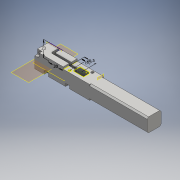
# Autodesk Inventor part: bas_de_fourche_gros_bloc
Saved by Autodesk Inventor 2016 (Build 200138000, 138)
## iProperties
Created: 2017-07-06
Part Number: bas_de_fourche_gros_bloc
Material: Generic
Document SubType Name: Modeling
Designer: mbouhier
Density: 1 g/cm^3
Appearance: Default
Author: mbouhier
Autodesk Inventor part; units mm, degrees
ref_plane "YZ Plane" through (0, 0, 0) normal (1, 0, 0) x (0, 1, 0)
ref_plane "XZ Plane" through (0, 0, 0) normal (0, 1, 0) x (-1, 0, 0)
ref_plane "XY Plane" through (0, 0, 0) normal (0, 0, 1) x (1, 0, 0)
sketch "Sketch1" plane through (0, 0, 0) normal (0, 1, 0) x (-1, 0, 0)
  line L0 (-10, 11.5) -> (10, 11.5)
  line L1 (10, 11.5) -> (10, -11.5)
  line L2 (10, -11.5) -> (-10, -11.5)
  line L3 (-10, -11.5) -> (-10, 11.5)
  line L4 (-10, 11.5) -> (10, -11.5) construction
  line L5 (10, 11.5) -> (-10, -11.5) construction
  point P0 (0, 0)
  dimension "d0" = 20
  dimension "d1" = 23
  constraints: 12 end point, 2 midpoint, 2 parallel, 1 horizontal, 1 perpendicular
  measures "d0" distance of L1.end L2.end
  measures "d1" distance of L0.end L1.end
extrude "Extrusion2" add sketch "Sketch1" against normal blind 20
ref_plane "Work Plane1" through (-10, 0, 0) normal (0, 0, 1) x (1, 0, 0)
ref_plane "Work Plane2" through (0, -2, 0) normal (0, 1, 0) x (1, 0, 0)
sketch "Sketch11" plane through (0, -2, 0) normal (0, 1, 0) x (1, 0, 0)
  point P0 (0, 0)
sketch "Sketch12" plane through (10, 0, 11.5) normal (1, 0, 0) x (0, 0, -1)
  line L0 (23, -20) -> (0, -20)
  line L1 (0, -20) -> (0, 0)
  line L2 (0, 0) -> (23, 0)
  line L3 (23, 0) -> (23, -20)
  point P0 (11.5, 0)
  dimension "d41" = 23
  dimension "d42" = 20
  constraints: 8 end point, 2 parallel, 1 horizontal, 1 perpendicular
  measures "d41" distance of L1.end L2.end
  measures "d42" distance of L0.end L1.end
extrude "Extrusion4" add sketch "Sketch12" along normal blind 22
sketch "Sketch13" plane through (32, 0, 11.5) normal (1, 0, 0) x (0, 0, -1)
  line L0 (23, 0) -> (23, -20) projected
  line L1 (23, -20) -> (3, -20)
  line L2 (3, -20) -> (3, 0)
  line L3 (3, 0) -> (23, 0)
  line L4 (23, 0) -> (23, -20)
  point P0 (11.5, 0)
  dimension "d45" = 20
  constraints: 8 end point, 2 parallel, 1 horizontal, 1 perpendicular
  measures "d45" distance of L1.end L2.end
extrude "Extrusion5" add sketch "Sketch13" along normal blind 120
sketch "Sketch26" plane through (32, -20, 8.5) normal (0, 0, 1) x (1, 0, 0)
  line L0 (8, 15) -> (23, 15)
  line L1 (23, 15) -> (23, 5)
  line L2 (23, 5) -> (8, 5)
  line L3 (8, 5) -> (8, 15)
  line L4 (0, 20) -> (120, 20) projected
  line L5 (0, 0) -> (120, 0) projected
  point P0 (-32, 20)
  dimension "d91" = 15
  dimension "d92" = 10
  dimension "d93" = 5
  dimension "d94" = 5
  constraints: 8 end point, 2 parallel, 1 horizontal, 1 perpendicular
  measures "d91" distance of L1.end L2.end
  measures "d92" distance of L0.end L1.end
  measures "d93" distance between parallel lines of L0 L4
  measures "d94" distance between parallel lines of L5 L2
extrude "Extrusion12" cut sketch "Sketch26" against normal blind 15
sketch "Sketch28" plane through (10, 0, -11.5) normal (0, 0, -1) x (-1, 0, 0)
  line L0 (-22, 0) -> (-22, -20) projected
  line L1 (20, -20) -> (-142, -20) projected
  line L2 (-22, 0) -> (-142, 0) projected
  point P0 (10, 0)
  point P1 (-27, -17)
  point P2 (-46, -3)
  dimension "d101" = 19
  dimension "d102" = 5
  dimension "d103" = 3
  dimension "d104" = 3
  measures "d101" horizontal distance of point (-46, -3) point (-27, -17)
  measures "d102" distance from line of L0 point (-27, -17)
  measures "d103" distance from line of L1 point (-27, -17)
  measures "d104" distance from line of L2 point (-46, -3)
hole "Hole3" at (56, -3, -11.5) at (37, -17, -11.5) direction (0, 0, 1) diameter 3.5 end through all counterbore diameter 5.5 counterbore depth 4
sketch "Sketch29" plane through (0, -20, 0) normal (0, -1, 0) x (1, 0, 0)
  line L0 (10, 11.5) -> (-10, 11.5) projected
  line L1 (10, -11.5) -> (10, 11.5) projected
  line L2 (-10, -11.5) -> (152, -11.5) projected
  line L3 (-10, 11.5) -> (-10, -11.5) projected
  point P0 (0, 0)
  point P1 (6.5, -8)
  point P2 (-6.5, 8)
  dimension "d112" = 3.5
  dimension "d113" = 3.5
  dimension "d128" = 3.5
  dimension "d129" = 3.5
  measures "d112" distance from line of L1 point (6.5, -8)
  measures "d113" distance from line of point (-6.5, 8) L3
  measures "d128" distance from line of L2 point (6.5, -8)
  measures "d129" distance from line of L0 point (-6.5, 8)
hole "Hole4" at (-6.5, -20, 8) at (6.5, -20, -8) direction (0, 1, 0) diameter 3.7 end through all counterbore diameter 6 counterbore depth 4
sketch "Sketch38" plane through (0, -20, 0) normal (0, -1, 0) x (1, 0, 0)
  circle A0 centre (-6.5, 8) radius 3 projected
  circle A1 centre (6.5, -8) radius 3 projected
  circle A2 centre (-6.5, 8) radius 3 projected
  circle A3 centre (6.5, -8) radius 3 projected
  line L0 (-10, 11.5) -> (32, 11.5) projected
  line L1 (-10, 11.5) -> (-10, -11.5) projected
  line L2 (-10, -11.5) -> (152, -11.5) projected
  line L3 (152, 8.5) -> (152, -11.5) projected
  line L4 (32, 8.5) -> (152, 8.5) projected
  line L5 (32, 11.5) -> (32, 8.5) projected
  circle A4 centre (-6.5, 8) radius 3 projected
  line L6 (-10, 11.5) -> (-10, -11.5) projected
  line L7 (-10, -11.5) -> (152, -11.5) projected
  line L8 (3.5, -11.5) -> (3.5, -8)
  circle A5 centre (6.5, -8) radius 3 projected
  line L9 (9.5, -8) -> (9.5, -11.5)
  line L10 (-3.5, 11.5) -> (-3.5, 8)
  line L11 (-10, 11.5) -> (-10, -11.5) projected
  line L12 (-10, 5) -> (-6.5, 5)
  point P0 (0, 0)
  constraints: 8 end point, 8 point on circle, 5 tangent, 4 point on line, 3 perpendicular, 1 parallel
extrude "Extrusion17" cut sketch "Sketch38" against normal up to surface (4 mm away) contours A0 L12 L1 L0 L10 | L8 A1 L9 L2
sketch "Sketch33" plane through (-10, -20, -11.5) normal (0, 0, -1) x (-1, 0, 0)
  circle A0 centre (-66, 17) radius 2.75
  circle A1 centre (-47, 3) radius 2.75
  line L0 (0, 20) -> (-162, 20)
  line L1 (0, 0) -> (-162, 0)
  circle A2 centre (-66, 17) radius 2.75
  line L2 (-63.25, 17) -> (-63.25, 20)
  line L3 (-68.749347, 16.940067) -> (-68.749347, 20)
  line L4 (-49.75, 3) -> (-49.75, 0)
  line L5 (-44.25, 3) -> (-44.25, 0)
  point P0 (-10, 20)
  constraints: 8 end point, 6 point on circle, 4 perpendicular, 4 point on line, 1 tangent
sketch "Sketch33 outline for Extrusion13" plane through (-10, -20, -11.5) normal (0, 0, -1) x (-1, 0, 0)
  arc A0 (-44.25, 3) -> (-49.75, 3) centre (-47, 3) cw
  line L0 (-44.25, 0) -> (-44.25, 3)
  line L1 (-49.75, 0) -> (-44.25, 0)
  line L2 (-49.75, 3) -> (-49.75, 0)
  arc A1 (-63.25, 17) -> (-68.749347, 17.059933) centre (-66, 17) ccw
  line L3 (-68.749347, 20) -> (-68.749347, 17.059933)
  line L4 (-63.25, 20) -> (-68.749347, 20)
  line L5 (-63.25, 17) -> (-63.25, 20)
extrude "Extrusion13" cut sketch "Sketch33 outline for Extrusion13" against normal up to surface (4 mm away)
sketch "Sketch34" plane through (32, 0, 11.5) normal (1, 0, 0) x (0, 0, -1)
  line L0 (3, -20) -> (3, 0) projected
  line L1 (3, 0) -> (0, 0) projected
  line L2 (0, 0) -> (0, -20) projected
  line L3 (0, -20) -> (3, -20) projected
  point P0 (11.5, 0)
extrude "ajustement" cut sketch "Sketch34" against normal blind 1
sketch "Sketch37" plane through (-10, -20, 11.5) normal (0, 0, 1) x (1, 0, 0)
  line L0 (20, 20) -> (20, 0) construction
  line L1 (0, 0) -> (41, 0) construction
  line L2 (20, 20) -> (40, 20) construction
  line L3 (50, 5) -> (50, 15) construction
  line L4 (50, 10) -> (20, 10) construction
  line L5 (50, 8.5) -> (17.5, 8.5)
  line L6 (17.5, 8.5) -> (14.5, 8.5)
  line L7 (14.5, 8.5) -> (14.5, 20)
  line L8 (41, 20) -> (0, 20) projected
  line L9 (50, 11.5) -> (17.5, 11.5)
  line L10 (17.5, 11.5) -> (17.5, 20)
  line L11 (17.5, 20) -> (14.5, 20)
  line L12 (50, 8.5) -> (50, 11.5)
  point P0 (10, 20)
  point P1 (20, 20)
  point P2 (0, 20)
  point P3 (17.5, 12)
  dimension "d137" = 90
  dimension "d138" = 2.5
  dimension "d139" = 1.5
  dimension "d140" = 1.5
  dimension "d141" = 3
  constraints: 20 end point, 4 horizontal, 4 point on line, 2 midpoint, 2 vertical, 1 collinear, 1 perpendicular, 3 other
  measures "d137" angle of L0 L2
  measures "d138" distance from line of point (17.5, 12) L0
  measures "d139" distance from line of L4 L9.start
  measures "d140" distance from line of L4 L5.start
  measures "d141" distance of L5.end L6.end
ref_plane "Work Plane4" through (-10, -20, -4.5) normal (0, 0, 1) x (1, 0, 0)
extrude "Extrusion16" cut sketch "Sketch37" against normal up to surface (16 mm away)
fillet "Fillet1" radius 2 4 edges at (4.5, -11.5, 3.5) (7.5, -8.5, 3.5) (40, -11.5, 2) (40, -8.5, 2)
fillet "Fillet2" radius 3 1 edges at (55, -5, 1)
sketch "Sketch39" plane through (152, -20, 8.5) normal (0, 0, 1) x (1, 0, 0)
  arc A0 (-97, 12) -> (-100, 15) centre (-100, 12) ccw projected
  line L0 (-112, 15) -> (-100, 15) projected
  line L1 (-112, 5) -> (-112, 15) projected
  line L2 (-97, 5) -> (-112, 5) projected
  line L3 (-97, 12) -> (-97, 5) projected
  line L4 (-121, 11.5) -> (-121, 20) projected
  circle A1 centre (-115, 3) radius 1.75 projected
  line L5 (-121, 0) -> (-121, 8.5) projected
  point P0 (-152, 20)
  point P1 (-104.5, 10)
  dimension "d149" = 16.5
  dimension "d150" = 6
  measures "d149" distance from line of point (-104.5, 10) L4
  measures "d150" distance from line of A1.centre L5
ref_plane "Work Plane5" through (69, 0, 11.5) normal (1, 0, 0) x (0, 0, -1)
sketch "Sketch41" plane through (152, 0, 11.5) normal (1, 0, 0) x (0, 0, -1)
  line L0 (3, -20) -> (23, -20) projected
  line L1 (23, -20) -> (23, 0) projected
  line L2 (23, 0) -> (3, 0) projected
  line L3 (3, 0) -> (3, -20) projected
  line L4 (3, -20) -> (23, -20) projected
  line L5 (5, -20) -> (3, -18)
  line L6 (21, -20) -> (23, -18)
  line L7 (23, -2) -> (21, 0)
  line L8 (23, 0) -> (3, 0) projected
  line L9 (5, 0) -> (3, -2)
  point P0 (11.5, 0)
  dimension "d152" = 2
  dimension "d153" = 2
  dimension "d154" = 2
  dimension "d155" = 2
  dimension "d156" = 2
  dimension "d157" = 2
  dimension "d158" = 2
  dimension "d159" = 2
  constraints: 10 point on line, 8 end point, 2 perpendicular
  measures "d152" distance of L0.start L5.start
  measures "d153" distance of L5.end L0.start
  measures "d154" distance of L2.end L9.end
  measures "d155" distance of L9.start L2.end
  measures "d156" distance of L1.end L7.end
  measures "d157" distance of L7.start L1.end
  measures "d158" distance of L0.end L6.start
  measures "d159" distance of L6.end L0.end
extrude "Extrusion18" cut sketch "Sketch41" against normal up to surface (83 mm away) contours L3 L5 L0 | L6 L1 L0 | L3 L2 L9 | L7 L2 L1
equation "\"d93\" = d94"
equation "\"d104\" = d103"
equation "\"d113\" = d112"
equation "\"d129\" = d128"
equation "\"d140\" = d139"
equation "\"d153\" = d152"
equation "\"d154\" = d152"
equation "\"d155\" = d152"
equation "\"d156\" = d152"
equation "\"d158\" = d152"
body "Solid1"
